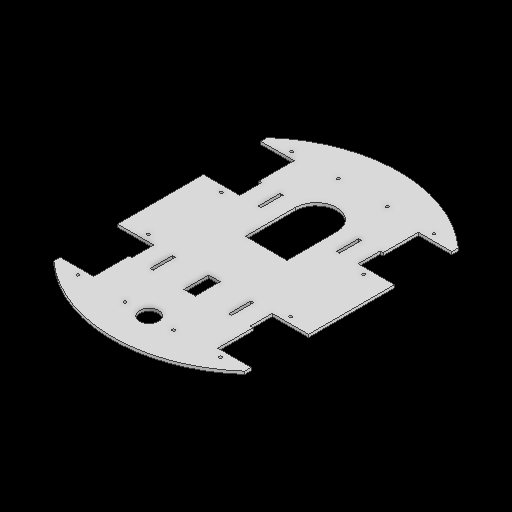
# Autodesk Inventor part: ChasisSuperior
Saved by Autodesk Inventor 2025.2 (Build 292293000, 293)
## iProperties
Created: 2024-12-02
Part Number: ChasisSuperior
Material: Generic
Document SubType Name: Modeling
Designer: braughton
Density: 1 g/cm^3
Appearance: Default
Author: braughton
Autodesk Inventor part; units mm, degrees
ref_plane "YZ Plane" through (0, 0, 0) normal (1, 0, 0) x (0, 1, 0)
ref_plane "XZ Plane" through (0, 0, 0) normal (0, 1, 0) x (-1, 0, 0)
ref_plane "XY Plane" through (0, 0, 0) normal (0, 0, 1) x (1, 0, 0)
sketch "Sketch1" plane through (0, 0, 0) normal (0, 1, 0) x (-1, 0, 0)
  circle A0 centre (225.7737, 188.8152) radius 1.5
  circle A1 centre (325.7737, 262.422) radius 1.5
  circle A2 centre (374.8449, 262.422) radius 1.5
  circle A3 centre (374.8449, 188.8152) radius 1.5
  circle A4 centre (274.8449, 38.8152) radius 1.5
  circle A5 centre (225.7737, 38.8152) radius 1.5
  circle A6 centre (225.7737, 112.422) radius 1.5
  circle A7 centre (325.7737, 38.8152) radius 1.5
  circle A8 centre (374.8449, 38.8152) radius 1.5
  circle A9 centre (374.8449, 112.422) radius 1.5
  line L0 (200.3093, 45.6186) -> (211.8093, 45.6186)
  line L1 (211.8093, 45.6186) -> (223.3093, 45.6186)
  line L2 (377.3093, 45.6186) -> (388.8093, 45.6186)
  line L3 (388.8093, 45.6186) -> (400.3093, 45.6186)
  line L4 (200.3093, 195.6186) -> (211.8093, 195.6186)
  line L5 (211.8093, 195.6186) -> (223.3093, 195.6186)
  line L6 (377.3093, 195.6186) -> (388.8093, 195.6186)
  line L7 (388.8093, 195.6186) -> (400.3093, 195.6186)
  line L8 (294.3093, 194.1186) -> (306.3093, 194.1186)
  line L9 (306.3093, 194.1186) -> (306.3093, 220.1186)
  line L10 (306.3093, 220.1186) -> (294.3093, 220.1186)
  line L11 (294.3093, 220.1186) -> (294.3093, 194.1186)
  arc A10 (278.5735, 87.7325) -> (322.2559, 87.7325) centre (300.4147, 87.7325) ccw
  circle A11 centre (300.4147, 262.422) radius 10
  line L12 (322.2559, 87.7325) -> (322.2559, 139.8246)
  line L13 (322.2559, 139.8246) -> (278.5735, 139.8246)
  line L14 (278.5735, 139.8246) -> (278.5735, 87.7325)
  circle A12 centre (274.8449, 262.422) radius 1.5
  circle A13 centre (225.7737, 262.422) radius 1.5
  line L15 (238.3093, 105.6186) -> (238.3093, 94.1186)
  line L16 (235.3093, 82.6186) -> (238.3093, 82.6186)
  line L17 (238.3093, 82.6186) -> (238.3093, 94.1186)
  line L18 (362.3093, 105.6186) -> (362.3093, 94.1186)
  line L19 (365.3093, 82.6186) -> (362.3093, 82.6186)
  line L20 (362.3093, 82.6186) -> (362.3093, 94.1186)
  line L21 (235.3093, 195.6186) -> (238.3093, 195.6186)
  line L22 (238.3093, 195.6186) -> (238.3093, 207.1186)
  line L23 (235.3093, 218.6186) -> (238.3093, 218.6186)
  line L24 (238.3093, 218.6186) -> (238.3093, 207.1186)
  line L25 (365.3093, 195.6186) -> (362.3093, 195.6186)
  line L26 (362.3093, 195.6186) -> (362.3093, 207.1186)
  line L27 (365.3093, 218.6186) -> (362.3093, 218.6186)
  line L28 (362.3093, 218.6186) -> (362.3093, 207.1186)
  line L29 (365.3093, 105.6186) -> (362.3093, 105.6186)
  arc A14 (300.3093, 0.6186) -> (400.3093, 38.8152) centre (300.3093, 150.6186) ccw
  arc A15 (200.3093, 38.8152) -> (300.3093, 0.6186) centre (300.3093, 150.6186) ccw
  line L30 (235.3093, 105.6186) -> (200.3093, 105.6186)
  line L31 (200.3093, 45.6186) -> (235.3093, 45.6186)
  line L32 (235.3093, 45.6186) -> (235.3093, 82.6186)
  arc A16 (300.3093, 300.6186) -> (200.3093, 262.422) centre (300.3093, 150.6186) ccw
  line L33 (235.3093, 195.6186) -> (200.3093, 195.6186)
  line L34 (200.3093, 255.6186) -> (235.3093, 255.6186)
  line L35 (235.3093, 255.6186) -> (235.3093, 218.6186)
  line L36 (365.3093, 105.6186) -> (400.3093, 105.6186)
  line L37 (400.3093, 45.6186) -> (365.3093, 45.6186)
  line L38 (365.3093, 45.6186) -> (365.3093, 82.6186)
  arc A17 (400.3093, 262.422) -> (300.3093, 300.6186) centre (300.3093, 150.6186) ccw
  line L39 (365.3093, 195.6186) -> (400.3093, 195.6186)
  line L40 (400.3093, 255.6186) -> (365.3093, 255.6186)
  line L41 (365.3093, 255.6186) -> (365.3093, 218.6186)
  line L42 (235.3093, 105.6186) -> (238.3093, 105.6186)
  line L43 (339.9093, 94.1186) -> (339.9093, 105.6186)
  line L44 (339.9093, 105.6186) -> (342.9093, 105.6186)
  line L45 (342.9093, 105.6186) -> (342.9093, 94.1186)
  line L46 (339.9093, 94.1186) -> (339.9093, 82.6186)
  line L47 (339.9093, 82.6186) -> (342.9093, 82.6186)
  line L48 (342.9093, 82.6186) -> (342.9093, 94.1186)
  line L49 (339.9093, 207.1186) -> (339.9093, 195.6186)
  line L50 (339.9093, 195.6186) -> (342.9093, 195.6186)
  line L51 (342.9093, 195.6186) -> (342.9093, 207.1186)
  line L52 (339.9093, 207.1186) -> (339.9093, 218.6186)
  line L53 (339.9093, 218.6186) -> (342.9093, 218.6186)
  line L54 (342.9093, 218.6186) -> (342.9093, 207.1186)
  line L55 (260.7093, 94.1186) -> (260.7093, 105.6186)
  line L56 (260.7093, 105.6186) -> (257.7093, 105.6186)
  line L57 (257.7093, 105.6186) -> (257.7093, 94.1186)
  line L58 (260.7093, 94.1186) -> (260.7093, 82.6186)
  line L59 (260.7093, 82.6186) -> (257.7093, 82.6186)
  line L60 (257.7093, 82.6186) -> (257.7093, 94.1186)
  line L61 (260.7093, 207.1186) -> (260.7093, 195.6186)
  line L62 (260.7093, 195.6186) -> (257.7093, 195.6186)
  line L63 (257.7093, 195.6186) -> (257.7093, 207.1186)
  line L64 (260.7093, 207.1186) -> (260.7093, 218.6186)
  line L65 (260.7093, 218.6186) -> (257.7093, 218.6186)
  line L66 (257.7093, 218.6186) -> (257.7093, 207.1186)
  line L67 (400.3093, 150.6186) -> (400.3093, 105.6186)
  line L68 (400.3093, 45.6186) -> (400.3093, 38.8152)
  line L69 (211.8093, 0.6186) -> (223.3093, 0.6186)
  line L70 (400.3093, 0.6186) -> (362.3093, 0.6186)
  line L71 (400.3093, 150.6186) -> (400.3093, 195.6186)
  line L72 (400.3093, 255.6186) -> (400.3093, 262.422)
  line L73 (200.3093, 150.6186) -> (200.3093, 195.6186)
  line L74 (200.3093, 150.6186) -> (200.3093, 195.6186)
  line L75 (200.3093, 255.6186) -> (200.3093, 262.422)
  line L76 (200.3093, 255.6186) -> (200.3093, 262.422)
  line L77 (200.3093, 150.6186) -> (200.3093, 105.6186)
  line L78 (200.3093, 45.6186) -> (200.3093, 38.8152)
  line L79 (200.3093, 150.6186) -> (200.3093, 105.6186)
  line L80 (200.3093, 45.6186) -> (200.3093, 38.8152)
  constraints: 162 end point, 18 centre point, 10 point on circle, 9 point on line
extrude "Extrusion1" add sketch "Sketch1" along normal blind 3
body "Solid1"
